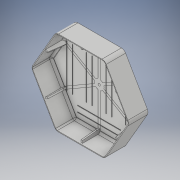
# Autodesk Inventor part: Base v5 - 175
Saved by Autodesk Inventor 2019 (Build 230136000, 136)
## iProperties
Created: 2021-07-14
Part Number: Base v5 - 175
Material: Generic
Document SubType Name: Modeling
Designer: Lix
Density: 1 g/cm^3
Appearance: Default
Author: Lix
## iProperties of the stored document Base v6 - 175_3DPrint.ipt
Created: 2021-08-07
Part Number: Base v6 - 175_3DPrint
Material: Generic
Document SubType Name: Modeling
Designer: Lix
Density: 1 g/cm^3
Appearance: Default
Author: Lix
Autodesk Inventor part; units mm, degrees
ref_plane "YZ Plane" through (0, 0, 0) normal (1, 0, 0) x (0, 1, 0)
ref_plane "XZ Plane" through (0, 0, 0) normal (0, 1, 0) x (-1, 0, 0)
ref_plane "XY Plane" through (0, 0, 0) normal (0, 0, 1) x (1, 0, 0)
sketch "Sketch1" plane through (0, 0, 0) normal (0, 0, 1) x (1, 0, 0)
  line L0 (50.5181, -87.5) -> (-50.5181, -87.5)
  line L1 (-50.5181, -87.5) -> (-101.0363, 0)
  line L2 (-101.0363, 0) -> (-50.5181, 87.5)
  line L3 (-50.5181, 87.5) -> (50.5181, 87.5)
  line L4 (50.5181, 87.5) -> (101.0363, 0)
  line L5 (101.0363, 0) -> (50.5181, -87.5)
  point P0 (0, 0)
  point P1 (0, 0)
  point P2 (0, 0)
  dimension "d0" = 175
  constraints: 12 end point, 2 coincident, 1 horizontal, 13 other
  measures "d0" distance between parallel lines of L5 L2
extrude "Extrusion1" add sketch "Sketch1" along normal blind 40
shell "Shell1" thickness 1.5 removed faces 1 at (16.8394, -29.1667, 40) ; own thickness 1 on faces at (16.8394, -29.1667, 0)
sketch "Sketch11" plane through (-49.6521, -86, 1) normal (0, 0, 1) x (1, 0, 0)
  line L0 (-16.5979, 42.5) -> (-5.5979, 42.5)
  line L1 (-5.5979, 42.5) -> (-5.5979, 129.5)
  line L2 (-5.5979, 129.5) -> (-16.5979, 129.5)
  line L3 (-16.5979, 129.5) -> (-16.5979, 42.5)
  line L4 (-16.5979, 42.5) -> (-5.5979, 129.5) construction
  line L5 (-5.5979, 42.5) -> (-16.5979, 129.5) construction
  line L6 (23.9021, 42.5) -> (34.9021, 42.5)
  line L7 (34.9021, 42.5) -> (34.9021, 129.5)
  line L8 (34.9021, 129.5) -> (23.9021, 129.5)
  line L9 (23.9021, 42.5) -> (34.9021, 129.5) construction
  line L10 (34.9021, 42.5) -> (23.9021, 129.5) construction
  line L11 (23.9021, 129.5) -> (23.9021, 42.5)
  line L12 (64.4021, 42.5) -> (75.4021, 42.5)
  line L13 (75.4021, 42.5) -> (75.4021, 129.5)
  line L14 (75.4021, 129.5) -> (64.4021, 129.5)
  line L15 (64.4021, 42.5) -> (75.4021, 129.5) construction
  line L16 (75.4021, 42.5) -> (64.4021, 129.5) construction
  line L17 (64.4021, 129.5) -> (64.4021, 42.5)
  line L18 (104.9021, 42.5) -> (115.9021, 42.5)
  line L19 (115.9021, 42.5) -> (115.9021, 129.5)
  line L20 (115.9021, 129.5) -> (104.9021, 129.5)
  line L21 (104.9021, 42.5) -> (115.9021, 129.5) construction
  line L22 (115.9021, 42.5) -> (104.9021, 129.5) construction
  line L23 (104.9021, 129.5) -> (104.9021, 42.5)
  line L24 (-11.0979, 86) -> (110.4021, 86) construction
  line L25 (6.1521, 15.5) -> (93.1521, 15.5)
  line L26 (93.1521, 15.5) -> (93.1521, 26.5)
  line L27 (93.1521, 26.5) -> (6.1521, 26.5)
  line L28 (6.1521, 26.5) -> (6.1521, 15.5)
  line L29 (6.1521, 15.5) -> (93.1521, 26.5) construction
  line L30 (93.1521, 15.5) -> (6.1521, 26.5) construction
  line L31 (49.6521, 21) -> (49.6521, 151) construction
  line L32 (6.1521, 145.5) -> (93.1521, 145.5)
  line L33 (93.1521, 145.5) -> (93.1521, 156.5)
  line L34 (93.1521, 156.5) -> (6.1521, 156.5)
  line L35 (6.1521, 156.5) -> (6.1521, 145.5)
  line L36 (6.1521, 145.5) -> (93.1521, 156.5) construction
  line L37 (93.1521, 145.5) -> (6.1521, 156.5) construction
  line L38 (5.1521, 157.5) -> (94.1521, 157.5)
  line L39 (94.1521, 157.5) -> (94.1521, 144.5)
  line L40 (94.1521, 144.5) -> (5.1521, 144.5)
  line L41 (5.1521, 144.5) -> (5.1521, 157.5)
  line L42 (-17.5979, 130.5) -> (-4.5979, 130.5)
  line L43 (-4.5979, 130.5) -> (-4.5979, 41.5)
  line L44 (-4.5979, 41.5) -> (-17.5979, 41.5)
  line L45 (-17.5979, 41.5) -> (-17.5979, 130.5)
  line L46 (22.9021, 130.5) -> (35.9021, 130.5)
  line L47 (35.9021, 130.5) -> (35.9021, 41.5)
  line L48 (35.9021, 41.5) -> (22.9021, 41.5)
  line L49 (22.9021, 41.5) -> (22.9021, 130.5)
  line L50 (63.4021, 130.5) -> (76.4021, 130.5)
  line L51 (76.4021, 130.5) -> (76.4021, 41.5)
  line L52 (76.4021, 41.5) -> (63.4021, 41.5)
  line L53 (63.4021, 41.5) -> (63.4021, 130.5)
  line L54 (103.9021, 130.5) -> (116.9021, 130.5)
  line L55 (116.9021, 130.5) -> (116.9021, 41.5)
  line L56 (116.9021, 41.5) -> (103.9021, 41.5)
  line L57 (103.9021, 41.5) -> (103.9021, 130.5)
  line L58 (94.1521, 14.5) -> (5.1521, 14.5)
  line L59 (5.1521, 14.5) -> (5.1521, 27.5)
  line L60 (5.1521, 27.5) -> (94.1521, 27.5)
  line L61 (94.1521, 27.5) -> (94.1521, 14.5)
  line L62 (115.9021, 130.5) -> (104.9021, 130.5)
  line L63 (104.9021, 130.5) -> (104.9021, 41.5)
  line L64 (104.9021, 41.5) -> (115.9021, 41.5)
  line L65 (115.9021, 41.5) -> (115.9021, 130.5)
  line L66 (75.4021, 130.5) -> (64.4021, 130.5)
  line L67 (64.4021, 130.5) -> (64.4021, 41.5)
  line L68 (64.4021, 41.5) -> (75.4021, 41.5)
  line L69 (75.4021, 41.5) -> (75.4021, 130.5)
  line L70 (94.1521, 156.5) -> (5.1521, 156.5)
  line L71 (5.1521, 156.5) -> (5.1521, 145.5)
  line L72 (5.1521, 145.5) -> (94.1521, 145.5)
  line L73 (94.1521, 145.5) -> (94.1521, 156.5)
  line L74 (-5.5979, 130.5) -> (-16.5979, 130.5)
  line L75 (-16.5979, 130.5) -> (-16.5979, 41.5)
  line L76 (-16.5979, 41.5) -> (-5.5979, 41.5)
  line L77 (-5.5979, 41.5) -> (-5.5979, 130.5)
  line L78 (34.9021, 130.5) -> (23.9021, 130.5)
  line L79 (23.9021, 130.5) -> (23.9021, 41.5)
  line L80 (23.9021, 41.5) -> (34.9021, 41.5)
  line L81 (34.9021, 41.5) -> (34.9021, 130.5)
  line L82 (94.1521, 26.5) -> (5.1521, 26.5)
  line L83 (5.1521, 26.5) -> (5.1521, 15.5)
  line L84 (5.1521, 15.5) -> (94.1521, 15.5)
  line L85 (94.1521, 15.5) -> (94.1521, 26.5)
  point P0 (49.6521, 86)
  point P1 (29.4021, 86)
  point P2 (69.9021, 86)
  point P3 (49.6521, 86)
  dimension "d138" = 11
  dimension "d139" = 87
  dimension "d142" = 40.5
  dimension "d147" = 130
  dimension "d151" = 1
  dimension "d152" = 1
  dimension "d153" = 1
  dimension "d154" = 1
  dimension "d155" = 1
  dimension "d156" = 1
  constraints: 172 end point, 24 parallel, 14 midpoint, 13 point on line, 12 perpendicular, 11 horizontal, 4 equal length, 1 coincident, 1 collinear, 1 horizontal alignment, 1 vertical, 50 other
  measures "d138" distance of L1.end L2.end
  measures "d139" distance of L2.end L0.start
  measures "d142" distance of L0.end L6.end
  measures "d147" distance of L31.start L31.end
  measures "d151" distance between parallel lines of L34 L38
  measures "d152" distance between parallel lines of L2 L42
  measures "d153" distance between parallel lines of L8 L46
  measures "d154" distance between parallel lines of L14 L50
  measures "d155" distance between parallel lines of L20 L54
  measures "d156" distance between parallel lines of L25 L58
extrude "Extrusion9" add sketch "Sketch11" along normal blind 0.5 contours L75 L44 L45 L42 L3 | L1 L77 L42 L43 L44 | L79 L48 L49 L46 L11 | L7 L81 L46 L47 L48 | L67 L52 L53 L50 L17 | L13 L69 L50 L51 L52 | L63 L56 L57 L54 L23 | L19 L65 L54 L55 L56 | L25 L84 L61 L58 L59 | L82 L59 L60 L61 L27 | L32 L72 L39 L40 L41 | L70 L41 L38 L39 L34
ref_plane "Work Plane1" through (-25.2591, 43.75, 40) normal (0.8660254, 0.5, 0) x (0, 0, -1)
ref_plane "Work Plane2" through (-50.5181, 0, 0) normal (0, 1, 0) x (1, 0, 0)
ref_plane "Work Plane3" through (-25.2591, -43.75, 0) normal (-0.8660254, 0.5, 0) x (0, 0, 1)
sketch "Sketch12" plane through (-49.6521, -86, 1) normal (0, 0, 1) x (1, 0, 0)
  line L0 (99.3042, 0) -> (0, 0) projected
  line L1 (148.9564, 86) -> (99.3042, 0) projected
  line L2 (99.3042, 172) -> (148.9564, 86) projected
  line L3 (0, 172) -> (99.3042, 172) projected
  line L4 (-49.6521, 86) -> (0, 172) projected
  line L5 (0, 0) -> (-49.6521, 86) projected
  point P0 (49.6521, 86)
sketch "Sketch4" plane through (-49.6521, -86, 1) normal (0, 0, 1) x (1, 0, 0)
  line L0 (99.3042, 0) -> (0, 0) projected
  line L1 (148.9564, 86) -> (99.3042, 0) projected
  line L2 (99.3042, 172) -> (148.9564, 86) projected
  line L3 (0, 172) -> (99.3042, 172) projected
  line L4 (-49.6521, 86) -> (0, 172) projected
  line L5 (0, 0) -> (-49.6521, 86) projected
  line L6 (-19.2831, 128.6007) -> (2.8868, 167)
  line L7 (2.8868, 167) -> (47.2265, 167)
  line L8 (99.3042, 172) -> (0, 0) construction
  arc A0 (47.2265, 95.7014) -> (42.4633, 92.9514) centre (49.6521, 86) ccw
  line L9 (-19.2831, 128.6007) -> (42.4633, 92.9514)
  line L10 (47.2265, 167) -> (47.2265, 95.7014)
  circle A1 centre (49.6521, 86) radius 2.5
  arc A2 (40.0377, 88.75) -> (40.0377, 83.25) centre (49.6521, 86) ccw
  line L11 (-21.7088, 124.3993) -> (40.0377, 88.75)
  line L12 (-21.7088, 47.6007) -> (40.0377, 83.25)
  line L13 (-21.7088, 47.6007) -> (-43.8786, 86)
  line L14 (-43.8786, 86) -> (-21.7088, 124.3993)
  arc A3 (42.4633, 79.0486) -> (47.2265, 76.2986) centre (49.6521, 86) ccw
  line L15 (-19.2831, 43.3993) -> (42.4633, 79.0486)
  line L16 (47.2265, 5) -> (47.2265, 76.2986)
  line L17 (47.2265, 5) -> (2.8868, 5)
  line L18 (2.8868, 5) -> (-19.2831, 43.3993)
  arc A4 (52.0778, 76.2986) -> (56.8409, 79.0486) centre (49.6521, 86) ccw
  line L19 (52.0778, 5) -> (52.0778, 76.2986)
  line L20 (118.5874, 43.3993) -> (56.8409, 79.0486)
  line L21 (118.5874, 43.3993) -> (96.4175, 5)
  line L22 (96.4175, 5) -> (52.0778, 5)
  arc A5 (59.2666, 83.25) -> (59.2666, 88.75) centre (49.6521, 86) ccw
  line L23 (121.013, 47.6007) -> (59.2666, 83.25)
  line L24 (121.013, 124.3993) -> (59.2666, 88.75)
  line L25 (121.013, 124.3993) -> (143.1829, 86)
  line L26 (143.1829, 86) -> (121.013, 47.6007)
  arc A6 (56.8409, 92.9514) -> (52.0778, 95.7014) centre (49.6521, 86) ccw
  line L27 (118.5874, 128.6007) -> (56.8409, 92.9514)
  line L28 (52.0778, 167) -> (52.0778, 95.7014)
  line L29 (52.0778, 167) -> (96.4175, 167)
  line L30 (96.4175, 167) -> (118.5874, 128.6007)
  point P0 (-49.6521, 86)
  point P1 (0, 0)
  point P2 (99.3042, 0)
  point P3 (148.9564, 86)
  point P4 (99.3042, 172)
  dimension "d37" = 5
  dimension "d44" = 10
  dimension "d45" = 60
  dimension "d46" = 90
  dimension "d47" = 90
  dimension "d52" = 5.5
  dimension "d55" = 5
  dimension "d72" = 360
  constraints: 50 end point, 12 point on circle, 7 centre point, 2 equal length, 1 coincident, 1 midpoint, 73 other
  measures "d37" distance between parallel lines of L3 L7
  measures "d44" radius of A0
  measures "d45" angle of L10 L9
  measures "d46" angle of L9 L6
  measures "d47" angle of L10 L7
  measures "d52" distance of L10.end L9.end
  measures "d55" diameter of A1
extrude "Extrusion5" cut sketch "Sketch4" against normal blind 0.01 contours L6 L7 L10 A0 L9 | A1 | A2 L12 L13 L14 L11 | A3 L16 L17 L18 L15 | A4 L20 L21 L22 L19 | A5 L24 L25 L26 L23 | A6 L28 L29 L30 L27
sketch "Sketch8" plane through (-49.6521, -86, 1) normal (0, 0, 1) x (1, 0, 0)
  line L0 (99.3042, 0) -> (0, 0) projected
  line L1 (148.9564, 86) -> (99.3042, 0) projected
  line L2 (99.3042, 172) -> (148.9564, 86) projected
  line L3 (0, 172) -> (99.3042, 172) projected
  line L4 (-49.6521, 86) -> (0, 172) projected
  line L5 (0, 0) -> (-49.6521, 86) projected
  line L6 (48.1521, 164) -> (51.1521, 164)
  line L7 (51.1521, 164) -> (51.1521, 172)
  line L8 (51.1521, 172) -> (48.1521, 172)
  line L9 (48.1521, 172) -> (48.1521, 164)
  line L10 (0, 172) -> (99.3042, 172) projected
  line L11 (49.6521, 86) -> (49.6521, 172)
  point P0 (49.6521, 86)
  point P1 (49.6521, 172)
  dimension "d57" = 3
  dimension "d58" = 8
  constraints: 10 end point, 2 midpoint, 2 parallel, 1 coincident, 1 collinear, 1 horizontal, 1 perpendicular, 1 vertical
  measures "d57" distance of L6.start L6.end
  measures "d58" distance of L6.end L7.end
extrude "Extrusion6" add sketch "Sketch8" along normal blind 36 contours L7 L6 L11 L3 | L3 L11 L6 L9
sketch "Sketch9" plane through (1.5, 78, 1) normal (1, 0, 0) x (0, 0, -1)
  line L0 (0, 0) -> (0, 8) projected
  line L1 (0, 0) -> (-36, 0) projected
  line L2 (-36, 8) -> (-36, 0) projected
  line L3 (0, 8) -> (-36, 8) projected
  line L4 (-36, 8) -> (-36, 0) projected
  line L5 (-36, 0) -> (-6, 0)
  line L6 (0, 0) -> (-36, 0) projected
  line L7 (-6, 0) -> (-36, 3)
  line L8 (-36, 3) -> (-36, 0)
  point P0 (1, -78)
  point P1 (-36, 8)
  dimension "d77" = 3
  dimension "d78" = 30
  constraints: 6 end point, 3 point on line, 1 collinear, 1 perpendicular
  measures "d77" distance of L7.end L5.start
  measures "d78" distance of L5.start L5.end
extrude "Extrusion8" cut sketch "Sketch9" against normal blind 20 contours L1 L2 L7
pattern_circular "Circular Pattern1" count 6 over 360 about axis through (0, 0, 1) along (0, 0, -1) of "Extrusion6", "Extrusion8"
fillet "Fillet1" radius 4 18 edges at (-25.5761, -86, 1) (25.5761, -86, 1) (-87.2662, -20.8505, 1) (-61.6902, -65.1495, 1) (61.6902, -65.1495, 1) (87.2662, -20.8505, 1) (87.2662, 20.8505, 1) (61.6902, 65.1495, 1) (25.5761, 86, 1) (-25.5761, 86, 1) (-61.6902, 65.1495, 1) (-87.2662, 20.8505, 1) (-99.3042, 0, 20.5) (-49.6521, 86, 20.5) (49.6521, 86, 20.5) (99.3042, 0, 20.5) (49.6521, -86, 20.5) (-49.6521, -86, 20.5)
fillet "Fillet2" radius 10 6 edges at (101.0363, 0, 20) (50.5181, 87.5, 20) (-50.5181, 87.5, 20) (50.5181, -87.5, 20) (-101.0363, 0, 20) (-50.5181, -87.5, 20)
fillet "Fillet4" radius 2 5 edges at (-7.1888, 6.9514, 0.995) (-2.4257, 9.7014, 0.995) (-2.4257, 81, 0.995) (-46.7654, 81, 0.995) (-68.9352, 42.6007, 0.995)
sketch "Sketch5" plane through (-44.7446, 87.5, 0) normal (0, 1, 0) x (1, 0, 0)
  line L0 (0, 0) -> (89.4893, 0) projected
  line L1 (0, -40) -> (0, 0) projected
  point P0 (44.7446, 0)
  point P1 (44.7446, -20)
  point P2 (44.7446, 0)
  point P3 (0, -20)
  constraints: 2 midpoint, 1 horizontal alignment, 1 vertical alignment
sketch "Sketch6" plane through (53.4049, 82.5, 40) normal (0.8660254, 0.5, 0) x (0, 0, -1)
  line L0 (40, 8.6603) -> (0, 8.6603) projected
  point P0 (40, -44.7446)
  point P1 (20, -44.7446)
  point P2 (20, 8.6603)
  constraints: 1 horizontal alignment, 1 midpoint, 1 vertical alignment
sketch "Sketch7" plane through (53.4049, -82.5, 40) normal (0.8660254, -0.5, 0) x (0, 0, -1)
  line L0 (0, -8.6603) -> (40, -8.6603) projected
  point P0 (40, 44.7446)
  point P1 (20, 44.7446)
  point P2 (20, -8.6603)
  constraints: 1 horizontal alignment, 1 midpoint, 1 vertical alignment
sketch "Sketch13" plane through (0, 0, 40) normal (0, 0, 1) x (1, 0, 0)
  line L0 (-66.25, -43.5) -> (-55.25, -43.5) projected
  line L1 (-55.25, -43.5) -> (-55.25, 43.5) projected
  line L2 (-55.25, 43.5) -> (-66.25, 43.5) projected
  line L3 (-66.25, 43.5) -> (-66.25, -43.5) projected
  line L4 (-25.75, -43.5) -> (-14.75, -43.5) projected
  line L5 (-14.75, -43.5) -> (-14.75, 43.5) projected
  line L6 (-14.75, 43.5) -> (-25.75, 43.5) projected
  line L7 (-25.75, 43.5) -> (-25.75, -43.5) projected
  line L8 (-43.5, 59.5) -> (43.5, 59.5) projected
  line L9 (43.5, 59.5) -> (43.5, 70.5) projected
  line L10 (43.5, 70.5) -> (-43.5, 70.5) projected
  line L11 (-43.5, 70.5) -> (-43.5, 59.5) projected
  line L12 (14.75, -43.5) -> (25.75, -43.5) projected
  line L13 (25.75, -43.5) -> (25.75, 43.5) projected
  line L14 (25.75, 43.5) -> (14.75, 43.5) projected
  line L15 (14.75, 43.5) -> (14.75, -43.5) projected
  line L16 (55.25, -43.5) -> (66.25, -43.5) projected
  line L17 (66.25, -43.5) -> (66.25, 43.5) projected
  line L18 (66.25, 43.5) -> (55.25, 43.5) projected
  line L19 (55.25, 43.5) -> (55.25, -43.5) projected
  line L20 (-43.5, -70.5) -> (43.5, -70.5) projected
  line L21 (43.5, -70.5) -> (43.5, -59.5) projected
  line L22 (43.5, -59.5) -> (-43.5, -59.5) projected
  line L23 (-43.5, -59.5) -> (-43.5, -70.5) projected
  arc A0 (-53.4049, -82.5) -> (-44.7446, -87.5) centre (-44.7446, -77.5) ccw projected
  line L24 (-44.7446, -87.5) -> (44.7446, -87.5) projected
  arc A1 (44.7446, -87.5) -> (53.4049, -82.5) centre (44.7446, -77.5) ccw projected
  line L25 (53.4049, -82.5) -> (98.1495, -5) projected
  arc A2 (98.1495, -5) -> (98.1495, 5) centre (89.4893, 0) ccw projected
  line L26 (98.1495, 5) -> (53.4049, 82.5) projected
  arc A3 (53.4049, 82.5) -> (44.7446, 87.5) centre (44.7446, 77.5) ccw projected
  line L27 (44.7446, 87.5) -> (-44.7446, 87.5) projected
  arc A4 (-44.7446, 87.5) -> (-53.4049, 82.5) centre (-44.7446, 77.5) ccw projected
  line L28 (-53.4049, 82.5) -> (-98.1495, 5) projected
  arc A5 (-98.1495, 5) -> (-98.1495, -5) centre (-89.4893, 0) ccw projected
  line L29 (-98.1495, -5) -> (-53.4049, -82.5) projected
  line L30 (-50.8068, -84) -> (-98.1495, -2) projected
  arc A6 (-98.1495, 2) -> (-98.1495, -2) centre (-94.6854, 0) ccw projected
  line L31 (-98.1495, 2) -> (-50.8068, 84) projected
  arc A7 (-47.3427, 86) -> (-50.8068, 84) centre (-47.3427, 82) ccw projected
  line L32 (-47.3427, 86) -> (47.3427, 86) projected
  arc A8 (50.8068, 84) -> (47.3427, 86) centre (47.3427, 82) ccw projected
  line L33 (50.8068, 84) -> (98.1495, 2) projected
  arc A9 (98.1495, -2) -> (98.1495, 2) centre (94.6854, 0) ccw projected
  line L34 (98.1495, -2) -> (50.8068, -84) projected
  arc A10 (47.3427, -86) -> (50.8068, -84) centre (47.3427, -82) ccw projected
  line L35 (47.3427, -86) -> (-47.3427, -86) projected
  arc A11 (-50.8068, -84) -> (-47.3427, -86) centre (-47.3427, -82) ccw projected
  line L36 (1.5, -81) -> (-1.5, -81) projected
  line L37 (-1.5, -81) -> (-1.5, -86) projected
  line L38 (1.5, -86) -> (-1.5, -86) projected
  line L39 (1.5, -86) -> (1.5, -81) projected
  line L40 (-69.3981, -41.799) -> (-70.8981, -39.201) projected
  line L41 (-70.8981, -39.201) -> (-75.2282, -41.701) projected
  line L42 (-73.7282, -44.299) -> (-75.2282, -41.701) projected
  line L43 (-73.7282, -44.299) -> (-69.3981, -41.799) projected
  line L44 (-66.8, -40.299) -> (-69.3981, -41.799) projected
  line L45 (-68.3, -37.701) -> (-66.8, -40.299) projected
  line L46 (-70.8981, -39.201) -> (-68.3, -37.701) projected
  line L47 (-69.3981, -41.799) -> (-70.8981, -39.201) projected
  line L48 (1.5, -78) -> (1.5, -81) projected
  line L49 (-1.5, -78) -> (1.5, -78) projected
  line L50 (-1.5, -81) -> (-1.5, -78) projected
  line L51 (1.5, -81) -> (-1.5, -81) projected
  line L52 (-70.8981, 39.201) -> (-69.3981, 41.799) projected
  line L53 (-69.3981, 41.799) -> (-73.7282, 44.299) projected
  line L54 (-75.2282, 41.701) -> (-73.7282, 44.299) projected
  line L55 (-75.2282, 41.701) -> (-70.8981, 39.201) projected
  line L56 (-68.3, 37.701) -> (-70.8981, 39.201) projected
  line L57 (-66.8, 40.299) -> (-68.3, 37.701) projected
  line L58 (-69.3981, 41.799) -> (-66.8, 40.299) projected
  line L59 (-70.8981, 39.201) -> (-69.3981, 41.799) projected
  line L60 (-1.5, 81) -> (1.5, 81) projected
  line L61 (1.5, 81) -> (1.5, 86) projected
  line L62 (-1.5, 86) -> (1.5, 86) projected
  line L63 (-1.5, 86) -> (-1.5, 81) projected
  line L64 (-1.5, 78) -> (-1.5, 81) projected
  line L65 (1.5, 78) -> (-1.5, 78) projected
  line L66 (1.5, 81) -> (1.5, 78) projected
  line L67 (-1.5, 81) -> (1.5, 81) projected
  line L68 (69.3981, 41.799) -> (70.8981, 39.201) projected
  line L69 (70.8981, 39.201) -> (75.2282, 41.701) projected
  line L70 (73.7282, 44.299) -> (75.2282, 41.701) projected
  line L71 (73.7282, 44.299) -> (69.3981, 41.799) projected
  line L72 (66.8, 40.299) -> (69.3981, 41.799) projected
  line L73 (68.3, 37.701) -> (66.8, 40.299) projected
  line L74 (70.8981, 39.201) -> (68.3, 37.701) projected
  line L75 (69.3981, 41.799) -> (70.8981, 39.201) projected
  line L76 (70.8981, -39.201) -> (69.3981, -41.799) projected
  line L77 (69.3981, -41.799) -> (73.7282, -44.299) projected
  line L78 (75.2282, -41.701) -> (73.7282, -44.299) projected
  line L79 (75.2282, -41.701) -> (70.8981, -39.201) projected
  line L80 (68.3, -37.701) -> (70.8981, -39.201) projected
  line L81 (66.8, -40.299) -> (68.3, -37.701) projected
  line L82 (69.3981, -41.799) -> (66.8, -40.299) projected
  line L83 (70.8981, -39.201) -> (69.3981, -41.799) projected
  point P0 (0, 0)
body "Solid1"
